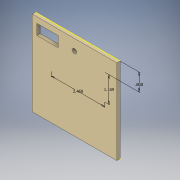
# Autodesk Inventor part: nEW bASE
Saved by Autodesk Inventor 2016 (Build 200138000, 138)
## iProperties
Created: 2017-09-12
Part Number: nEW bASE
Material: Generic
Document SubType Name: Modeling
Designer: student
Density: 1 g/cm^3
Appearance: Default
Author: student
Autodesk Inventor part; units mm, degrees
ref_plane "YZ Plane" through (0, 0, 0) normal (1, 0, 0) x (0, 1, 0)
ref_plane "XZ Plane" through (0, 0, 0) normal (0, 1, 0) x (-1, 0, 0)
ref_plane "XY Plane" through (0, 0, 0) normal (0, 0, 1) x (1, 0, 0)
sketch "Sketch1" plane through (0, 0, 0) normal (0, 0, 1) x (1, 0, 0)
  line L0 (0, 0) -> (-99.06, 0)
  line L1 (-99.06, 0) -> (-99.06, 99.06)
  line L2 (-99.06, 99.06) -> (0, 99.06)
  line L3 (0, 99.06) -> (0, 0)
  circle A0 centre (-49.53, 86.3053) radius 2.54
  line L4 (-93.595, 80.1839) -> (-68.5299, 80.1839)
  line L5 (-68.5299, 80.1839) -> (-68.5299, 92.4267)
  line L6 (-68.5299, 92.4267) -> (-93.595, 92.4267)
  line L7 (-93.595, 92.4267) -> (-93.595, 80.1839)
  dimension "d0" = 99.06
  dimension "d1" = 99.06
  dimension "d2" = 5.08
  constraints: 16 end point, 4 parallel, 2 horizontal, 2 perpendicular, 1 centre point
  measures "d0" distance of L1.end L2.end
  measures "d1" distance of L0.end L1.end
  measures "d2" diameter of A0
extrude "Extrusion1" add sketch "Sketch1" along normal blind 3.81
sketch "Sketch2" plane through (0, 0, 0) normal (0, 0, -1) x (-1, 0, 0)
  line L0 (0, 0) -> (99.06, 0) projected
  line L1 (99.06, 0) -> (99.06, 99.06) projected
  line L2 (50.116, 24.3723) -> (61.165, 24.3723)
  line L3 (61.165, 24.3723) -> (61.165, 46.3433)
  line L4 (61.165, 46.3433) -> (50.116, 46.3433)
  line L5 (50.116, 46.3433) -> (50.116, 24.3723)
  line L6 (48.9458, 24.3707) -> (37.8968, 24.3707)
  line L7 (37.8968, 24.3707) -> (37.8968, 46.3417)
  line L8 (37.8968, 46.3417) -> (48.9458, 46.3417)
  line L9 (48.9458, 46.3417) -> (48.9458, 24.3707)
  line L10 (50.116, 46.3433) -> (48.7841, 46.3433) construction
  dimension "d5" = 11.049
  dimension "d6" = 21.971
  dimension "d8" = 11.049
  dimension "d9" = 21.971
  constraints: 18 end point, 4 parallel, 3 horizontal, 2 perpendicular
  measures "d5" distance of L4.end L3.end
  measures "d6" distance of L3.end L2.end
  measures "d8" distance of L7.end L8.end
  measures "d9" distance of L6.end L7.end
extrude "Extrusion2" add sketch "Sketch2" along normal blind 8.89
sketch "Sketch3" plane through (0, 0, 0) normal (0, 0, -1) x (-1, 0, 0)
  line L0 (80.5561, 78.74) -> (17.8689, 78.74)
  line L1 (17.8689, 78.74) -> (17.8689, 48.5394)
  line L2 (17.8689, 48.5394) -> (80.5561, 48.5394)
  line L3 (80.5561, 48.5394) -> (80.5561, 78.74)
  line L4 (80.5561, 78.74) -> (17.8689, 48.5394) construction
  line L5 (17.8689, 78.74) -> (80.5561, 48.5394) construction
  line L6 (99.06, 99.06) -> (0, 99.06) projected
  point P0 (0, 0)
  point P1 (49.2125, 63.6397)
  dimension "d12" = 62.6872
  dimension "d13" = 30.2006
  dimension "d14" = 20.32
  constraints: 12 end point, 2 midpoint, 2 parallel, 1 horizontal, 1 perpendicular
  measures "d12" distance of L2.end L1.end
  measures "d13" distance of L1.end L0.end
  measures "d14" distance between parallel lines of L6 L0
body "Solid1"
